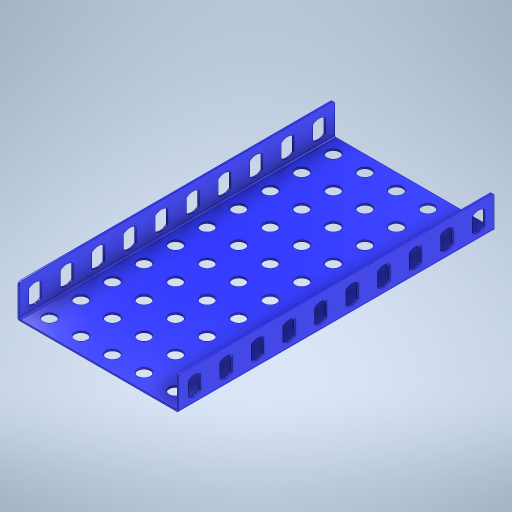
# Autodesk Inventor part: 1036
Saved by Autodesk Inventor 2024 (Build 280153000, 153)
## iProperties
Created: 2024-09-13
Part Number: 1036
Material: Všeobecné
Document SubType Name: Modeling
Designer: Student
Density: 1 g/cm^3
Appearance: Modrá – nástěnná malba – lesklá
Author: Student
Autodesk Inventor part; units mm, degrees
ref_plane "XZ Plane" through (0, 0, 0) normal (0, 1, 0) x (-1, 0, 0)
ref_plane "XY Plane" through (0, 0, 0) normal (0, 0, 1) x (1, 0, 0)
sketch "Náčrt1" plane through (0, 0, 0) normal (0, 0, 1) x (1, 0, 0)
  line L0 (-24.5, 0.5) -> (24.5, 0.5)
  line L1 (25, 1) -> (25, 10.5)
  line L2 (25, 10.5) -> (25.5, 10.5)
  line L3 (25.5, 10.5) -> (25.5, 0.5)
  line L4 (25, 0) -> (-25, 0)
  line L5 (-25.5, 0.5) -> (-25.5, 10.5)
  line L6 (-25.5, 10.5) -> (-25, 10.5)
  line L7 (-25, 10.5) -> (-25, 1)
  arc A0 (25, 0) -> (25.5, 0.5) centre (25, 0.5) ccw
  arc A1 (-25.5, 0.5) -> (-25, 0) centre (-25, 0.5) ccw
  arc A2 (24.5, 0.5) -> (25, 1) centre (24.5, 1) ccw
  arc A3 (-25, 1) -> (-24.5, 0.5) centre (-24.5, 1) ccw
  point P0 (0, 0)
  point P1 (-25, 0.5)
  point P2 (25, 0.5)
  point P3 (25.5, 0)
  point P4 (-25.5, 0)
  point P5 (25.5, 5.5)
  point P6 (25, 5.75)
  point P7 (-25.5, 5.5)
  point P8 (-25, 5.75)
  dimension "d0" = 51
  dimension "d1" = 25.5
  dimension "d2" = 0.5
  dimension "d3" = 0.5
  dimension "d4" = 0.5
  dimension "d7" = 10
  dimension "d34" = 0.5
  dimension "d35" = 0.5
  constraints: 16 end point, 10 point on line, 8 point on circle, 8 tangent, 6 perpendicular, 4 centre point, 4 midpoint, 2 equal radius, 1 horizontal
  measures "d0" distance of point (25.5, 0) point (-25.5, 0)
  measures "d1" horizontal distance of L2.end point (0, 0)
  measures "d2" horizontal distance of point (25.5, 5.5) point (25, 5.75)
  measures "d3" distance between parallel lines of L4 L0
  measures "d4" horizontal distance of point (-25.5, 5.5) point (-25, 5.75)
  measures "d7" distance from line of L1.end L0
  measures "d34" radius of A0
  measures "d35" radius of A2
extrude "Vysunutí1" add sketch "Náčrt1" along normal blind 100
sketch "Náčrt2" plane through (0, 0, 0) normal (0, 1, 0) x (-1, 0, 0)
  circle A0 centre (20.5, 5) radius 2
  line L0 (25.5, 0) -> (25.5, 50) projected
  line L1 (25, 0) -> (-25, 0) projected
  point P0 (0, 0)
  point P1 (-25.5, 0)
  dimension "d8" = 4
  dimension "d9" = 5
  dimension "d10" = 5
  constraints: 1 centre point
  measures "d8" diameter of A0
  measures "d9" distance from line of A0.centre L0
  measures "d10" distance from line of L1 A0.centre
extrude "Vysunutí2" cut sketch "Náčrt2" along normal through all
pattern_linear "Obdélníkové pole1" count 5 spacing 10 along (1, 0, 0) count 10 spacing 10 along (0, 0, 1) of "Vysunutí2"
ref_plane "Pracovní rovina1" through (-25.5, 0, 0) normal (1, 0, 0) x (0, 1, 0)
sketch "Náčrt4" plane through (-25.5, 0, 0) normal (1, 0, 0) x (0, 1, 0)
  line L0 (10.5, 0) -> (0, 0) projected
  line L1 (0, 0) -> (0, 50) projected
  line L2 (2, 7) -> (8, 7)
  line L3 (2, 3) -> (8, 3)
  arc A0 (7.2361, 3) -> (7.2361, 7) centre (5, 5) ccw
  arc A1 (2.7639, 7) -> (2.7639, 3) centre (5, 5) ccw
  dimension "d21" = 5
  dimension "d22" = 5
  dimension "d23" = 6
  dimension "d24" = 4
  dimension "d25" = 2
  dimension "d26" = 6
  dimension "d27" = 3
  dimension "d28" = 3
  constraints: 4 end point, 4 point on circle, 4 point on line, 2 centre point, 2 horizontal
  measures "d21" distance from line of L0 A0.centre
  measures "d22" distance from line of L1 A0.centre
  measures "d23" distance of L2.start L2.end
  measures "d24" distance between parallel lines of L3 L2
  measures "d25" distance from line of L3 A0.centre
  measures "d26" distance of L3.start L3.end
  measures "d27" horizontal distance of A0.centre L2.start
  measures "d28" horizontal distance of A0.centre L3.end
extrude "Vysunutí3" cut sketch "Náčrt4" along normal through all
pattern_linear "Obdélníkové pole2" count 10 spacing 10 along (0, 0, 1) of "Vysunutí3"
fillet "Zaoblení1" radius 1 2 edges at (-25.25, 10.5, 100) (25.25, 10.5, 100)
fillet "Zaoblení2" radius 1 2 edges at (25.25, 10.5, 0) (-25.25, 10.5, 0)
equation "\"d1\" = 0.5 * d0"
